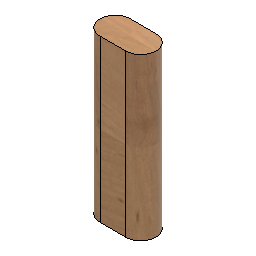
Connector set EV-32 Set Configurable (Autodesk Fusion 360 archive; units mm, degrees)
design "14x75"
description: Festool Domino
part number: 14x75
Autodesk Fusion 360 part; units mm, degrees
sketch "Sketch1" plane through (0, 0, 0) normal (0, 1, 0) x (1, 0, 0)
  line L0 (-6, -7) -> (6, -7)
  arc A0 (6, -7) -> (6, 7) centre (6, 0) ccw
  line L1 (6, 7) -> (-6, 7)
  arc A1 (-6, 7) -> (-6, -7) centre (-6, 0) ccw
  line L2 (-6, 0) -> (6, 0) construction
  dimension "d4" = 6
  dimension "d5" = 14
  constraint tangent L0 A0
  constraint tangent A0 L1
  constraint parallel L0 L1
  constraint tangent L1 A1
  constraint tangent L0 A1
  constraint horizontal L2
  constraint midpoint L2 origin
  measures "d4" distance of origin A0.centre
  measures "d5" distance of L0 L1
extrude "Extrude1" add sketch "Sketch1" along normal mid plane 75 makes body 1
extrude "Extrude2" add sketch "Sketch1" along normal mid plane 81 separate body makes body 2
hidden bodies 2
equation "Length = 75 mm"
equation "Thickness = 14 mm"
equation "Width = 12 mm"
equation "d4 = Width / 2"
equation "d5 = Thickness"
equation "d6 = Length"
equation "d8 = Length + 6 mm"
named bodies: "Domino", "Hole"

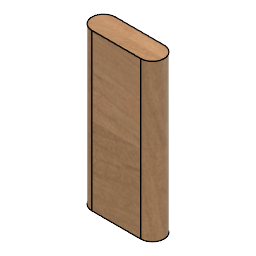
design "Festool Domino"
description: Festool Domino
part number: 6x40
Autodesk Fusion 360 part; units mm, degrees
sketch "Sketch1" plane through (0, 0, 0) normal (0, 1, 0) x (1, 0, 0)
  line L0 (-6.25, -3) -> (6.25, -3)
  arc A0 (6.25, -3) -> (6.25, 3) centre (6.25, 0) ccw
  line L1 (6.25, 3) -> (-6.25, 3)
  arc A1 (-6.25, 3) -> (-6.25, -3) centre (-6.25, 0) ccw
  line L2 (-6.25, 0) -> (6.25, 0) construction
  dimension "d4" = 6.25
  dimension "d5" = 6
  constraint tangent L0 A0
  constraint tangent A0 L1
  constraint parallel L0 L1
  constraint tangent L1 A1
  constraint tangent L0 A1
  constraint horizontal L2
  constraint midpoint L2 origin
  measures "d4" distance of origin A0.centre
  measures "d5" distance of L0 L1
extrude "Extrude1" add sketch "Sketch1" along normal mid plane 40 makes body 1
extrude "Extrude2" add sketch "Sketch1" along normal mid plane 46 separate body makes body 2
hidden bodies 2
equation "Length = 40 mm"
equation "Thickness = 6 mm"
equation "Width = 12.5 mm"
equation "d4 = Width / 2"
equation "d5 = Thickness"
equation "d6 = Length"
equation "d8 = Length + 6 mm"
named bodies: "Domino", "Hole"
